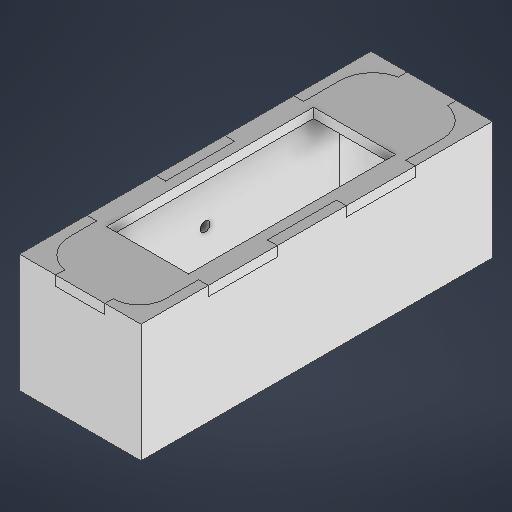
# Autodesk Inventor part: camerahouse
Saved by Autodesk Inventor 2026.2 (Build 302298000, 298)
## iProperties
Created: 2026-02-10
Part Number: camerahouse
Material: Generic
Document SubType Name: Modeling
Designer: small.ab
Density: 1 g/cm^3
Appearance: Default
Author: small.ab
Autodesk Inventor part; units mm, degrees
ref_plane "YZ Plane" through (0, 0, 0) normal (1, 0, 0) x (0, 1, 0)
ref_plane "XZ Plane" through (0, 0, 0) normal (0, 1, 0) x (-1, 0, 0)
ref_plane "XY Plane" through (0, 0, 0) normal (0, 0, 1) x (1, 0, 0)
sketch "Sketch1" plane through (0, 0, 0) normal (0, 0, 1) x (1, 0, 0)
  line L0 (0, 0) -> (100, 0)
  line L1 (100, 0) -> (100, 25)
  line L2 (100, 25) -> (0, 25)
  line L3 (0, 25) -> (0, 0)
  dimension "cameralength" = 100
  dimension "cameraheight" = 25
  constraints: 8 end point, 2 parallel, 1 horizontal, 1 perpendicular
  measures "cameralength" distance of L2.end L1.end
  measures "cameraheight" distance of L0.end L1.end
extrude "Extrusion1" add sketch "Sketch1" along normal blind 30
sketch "Sketch2" plane through (0, 0, 0) normal (0, -1, 0) x (1, 0, 0)
  line L0 (0, 0) -> (0, 30) projected
  line L1 (100, 30) -> (0, 30) projected
  line L2 (100, 0) -> (100, 30) projected
  circle A0 centre (49.9989, 14.9997) radius 9.6139
  dimension "bottomdiameter" = 19.2278
  constraints: 1 centre point
  measures "bottomdiameter" diameter of A0
extrude "Extrusion2" add sketch "Sketch2" along normal blind 5
fillet "Fillet1" radius 10 4 edges at (100, 0, 15) (100, 25, 15) (0, 0, 15) (0, 25, 15)
sketch "Sketch3" plane through (49.9989, 25, 30) normal (0, 0, 1) x (1, 0, 0)
  line L0 (53.5011, -33.5) -> (-53.4989, -33.5)
  line L1 (-53.4989, -33.5) -> (-53.4989, 3.5)
  line L2 (-53.4989, 3.5) -> (53.5011, 3.5)
  line L3 (53.5011, 3.5) -> (53.5011, -33.5)
  line L4 (53.5011, -33.5) -> (-53.4989, 3.5) construction
  line L5 (-53.4989, -33.5) -> (53.5011, 3.5) construction
  line L6 (50.0011, -25) -> (50.0011, -25) projected
  line L7 (-49.9989, -25) -> (50.0011, -25) projected
  line L8 (-49.9989, -25) -> (50.0011, -25) projected
  line L9 (50.0011, -25) -> (50.0011, -25) projected
  line L10 (-49.9989, -25) -> (50.0011, -25) projected
  line L11 (-49.9989, -25) -> (-49.9989, -25) projected
  line L12 (-42.9989, 0.5) -> (41.0011, 0.5)
  line L13 (51.0011, -9.5) -> (51.0011, -20.5)
  line L14 (41.0011, -30.5) -> (-40.9989, -30.5)
  line L15 (-50.9989, -20.5) -> (-50.9989, -7.5)
  line L16 (-50.9989, 0.5) -> (51.0011, -30.5) construction
  line L17 (51.0011, 0.5) -> (-50.9989, -30.5) construction
  line L18 (50.0011, -25) -> (50.0011, 0) projected
  line L19 (-9.6139, -30) -> (9.6139, -30) projected
  line L20 (9.6139, -25) -> (-9.6139, -25) projected
  line L21 (50.0011, 0) -> (-49.9989, 0) projected
  arc A0 (-50.9989, -20.5) -> (-40.9989, -30.5) centre (-40.9989, -20.5) ccw
  arc A1 (-42.9989, 0.5) -> (-50.9989, -7.5) centre (-42.9989, -7.5) ccw
  arc A2 (41.0011, -30.5) -> (51.0011, -20.5) centre (41.0011, -20.5) ccw
  arc A3 (51.0011, -9.5) -> (41.0011, 0.5) centre (41.0011, -9.5) ccw
  point P0 (0.0011, -15)
  point P1 (50.0011, 15.0003)
  point P2 (-49.9989, -14.9997)
  point P3 (44.1236, 0)
  point P4 (50.0011, -5.1411)
  point P5 (50.0011, -24.8589)
  point P6 (49.9314, -25)
  dimension "d7" = 37
  dimension "d8" = 107
  dimension "d9" = 3.5
  dimension "d16" = 1
  dimension "d18" = 0.5
  dimension "d19" = 31
  dimension "d20" = 3
  dimension "fillet" = 10
  dimension "d25" = 8
  dimension "d26" = 10
  dimension "d27" = 10
  constraints: 24 end point, 8 point on circle, 8 point on line, 8 tangent, 4 centre point, 4 midpoint, 4 parallel, 2 horizontal, 2 perpendicular
  measures "d7" distance between parallel lines of L0 L2
  measures "d8" distance between parallel lines of L3 L1
  measures "d9" distance between parallel lines of L3 L6
  measures "d16" distance between parallel lines of L13 L18
  measures "d18" distance between parallel lines of L12 L21
  measures "d19" distance between parallel lines of L12 L14
  measures "d20" distance between parallel lines of L14 L0
  measures "fillet" radius of A0
  measures "d25" radius of A1
  measures "d26" radius of A2
  measures "d27" radius of A3
extrude "Extrusion3" add sketch "Sketch3" against normal blind 33 separate body contours L0 L1 L2 L3 | A3 L21 L18
sketch "Sketch4" plane through (49.9989, 25, 30) normal (0, 0, 1) x (1, 0, 0)
  line L0 (53.5011, 3.5) -> (-53.4989, 3.5) projected
  line L1 (-53.4989, 3.5) -> (-53.4989, -33.5) projected
  line L2 (-53.4989, -33.5) -> (53.5011, -33.5) projected
  line L3 (53.5011, -33.5) -> (53.5011, 3.5) projected
  line L4 (-42.9989, 0.5) -> (41.0011, 0.5) projected
  line L5 (51.0011, -9.5) -> (51.0011, -20.5) projected
  line L6 (41.0011, -30.5) -> (-40.9989, -30.5) projected
  line L7 (-50.9989, -20.5) -> (-50.9989, -7.5) projected
  line L8 (-53.4989, 3.5) -> (53.5011, 3.5)
  line L9 (53.5011, 3.5) -> (53.5011, -33.5)
  line L10 (53.5011, -33.5) -> (-53.4989, -33.5)
  line L11 (-53.4989, -33.5) -> (-53.4989, 3.5)
  circle A0 centre (0.0011, -12.5) radius 10
  line L12 (50.0011, -15) -> (50.0011, -10) projected
  line L13 (40.0011, 0) -> (-39.9989, 0) projected
  line L14 (-49.9989, -10) -> (-49.9989, -15) projected
  line L15 (-39.9989, -25) -> (40.0011, -25) projected
  arc A1 (51.0011, -9.5) -> (41.0011, 0.5) centre (41.0011, -9.5) ccw projected
  line L16 (50.0011, -24.8589) -> (50.0011, -25) projected
  arc A2 (50.0011, -24.8589) -> (51.0011, -20.5) centre (41.0011, -20.5) ccw projected
  line L17 (50.0011, -25) -> (49.9314, -25) projected
  arc A3 (41.0011, -30.5) -> (49.9314, -25) centre (41.0011, -20.5) ccw projected
  arc A4 (-50.9989, -20.5) -> (-40.9989, -30.5) centre (-40.9989, -20.5) ccw projected
  arc A5 (-42.9989, 0.5) -> (-50.9989, -7.5) centre (-42.9989, -7.5) ccw projected
  arc A6 (-39.9989, 0) -> (-49.9989, -10) centre (-39.9989, -10) ccw projected
  arc A7 (-49.9989, -15) -> (-39.9989, -25) centre (-39.9989, -15) ccw projected
  arc A8 (40.0011, -25) -> (50.0011, -15) centre (40.0011, -15) ccw projected
  arc A9 (50.0011, -10) -> (40.0011, 0) centre (40.0011, -10) ccw projected
  point P0 (-49.9989, -25)
  dimension "cordhole" = 20
  constraints: 8 end point, 2 parallel, 1 centre point, 1 horizontal, 1 perpendicular
  measures "cordhole" diameter of A0
extrude "Extrusion4" add sketch "Sketch4" along normal blind 3 contours L3 L2 L1 L0 | L4 A1 L5 A2 L16 L17 A3 L6 A4 L7 A5 | A8 L15 A7 L14 A6 L13 A9 L12 bodies 2
sketch "Sketch5" plane through (-3.5, -8.5, 0) normal (0, -1, 0) x (1, 0, 0)
  circle A0 centre (53.4989, 14.9997) radius 9.6139 projected
  circle A1 centre (53.4989, 14.9997) radius 1.5
  point P0 (3.5, 0)
  dimension "screwdiameter" = 3
  constraints: 1 centre point, 1 coincident
  measures "screwdiameter" diameter of A1
extrude "Extrusion5" cut sketch "Sketch5" against normal blind 3 contours A1 bodies 2
sketch "Sketch7" plane through (-3.5, 28.5, 0) normal (0, 1, 0) x (1, 0, 0)
  line L0 (0, 3) -> (0, -33) projected
  line L1 (107, -33) -> (0, -33) projected
  line L2 (107, -33) -> (107, 3) projected
  line L3 (104.5, -30) -> (104.5, 3) projected
  line L4 (2.5, -30) -> (2.5, 3) projected
  line L5 (104.5, 0) -> (2.5, 0)
  line L6 (2.5, 0) -> (2.5, 0)
  line L7 (2.5, 0) -> (104.5, 0)
  line L8 (104.5, 0) -> (104.5, 0)
  line L9 (83.5, 0) -> (83.5, 0)
  line L10 (62.5, 0) -> (62.5, 0)
  line L11 (41.5, -3) -> (41.5, 0)
  line L12 (20.5, -3) -> (20.5, 0)
  line L13 (0, 3) -> (107, 3) projected
  line L14 (83.5, 0) -> (83.5, 3)
  line L15 (62.5, 0) -> (62.5, 3)
  line L16 (41.5, 0) -> (41.5, 3)
  line L17 (20.5, 0) -> (20.5, 3)
  line L18 (0, 3) -> (107, 3) projected
  point P0 (3.5, 0)
  point P1 (20.5, 0)
  point P2 (41.5, 0)
  point P3 (62.5, -3)
  point P4 (20.5, 0)
  point P5 (62.5, 0)
  point P6 (41.5, 0)
  point P7 (20.5, 0)
  point P8 (41.5, 0)
  dimension "d44" = 21
  dimension "d47" = 21
  dimension "d59" = 3
  constraints: 24 end point, 7 point on line, 5 perpendicular, 2 equal length, 1 horizontal
  measures "d44" distance between parallel lines of L9 L3
  measures "d47" distance of L9.start L10.start
  measures "d59" distance between parallel lines of L13 L7
extrude "Extrusion9" cut sketch "Sketch7" against normal up to surface (37 mm away) contours L13 L16 L5 L17 | L13 L14 L5 L15 bodies 2
sketch "Sketch8" plane through (103.5, -8.5, 0) normal (1, 0, 0) x (0, 0, -1)
  line L0 (-33, 37) -> (3, 37) projected
  line L1 (-33, 0) -> (-33, 37) projected
  line L2 (3, 0) -> (-33, 0) projected
  line L3 (-30, 3) -> (3, 3) projected
  line L4 (-30, 34) -> (3, 34) projected
  line L5 (3, 37) -> (3, 0) projected
  line L6 (3, 37) -> (0, 37)
  line L7 (0, 37) -> (0, 0)
  line L8 (0, 0) -> (3, 0)
  line L9 (3, 0) -> (3, 37)
  line L10 (0, 26) -> (3, 26)
  line L11 (0, 11) -> (3, 11)
  line L12 (3, 13) -> (3, 8.6411) projected
  point P0 (-3, 34)
  point P1 (0, 3)
  dimension "d62" = 11
  dimension "d63" = 11
  constraints: 12 end point, 5 point on line, 3 parallel, 2 perpendicular, 1 horizontal
  measures "d62" distance between parallel lines of L2 L11
  measures "d63" distance from line of L10 L0.end
extrude "Extrusion10" cut sketch "Sketch8" against normal up to surface (107 mm away) contours L10 L5 L11 L7 bodies 2
sketch "Sketch11" plane through (49.9989, 25, -3) normal (0, 0, -1) x (-1, 0, 0)
  line L0 (-53.5011, -7.5) -> (-50.7991, -7.5) projected
  arc A0 (-41.0011, 0.5) -> (-50.7991, -7.5) centre (-41.0011, -9.5) ccw projected
  line L1 (-41.0011, 0.5) -> (-30.0011, 0.5) projected
  line L2 (-30.0011, 0.5) -> (-30.0011, 3.5) projected
  line L3 (-30.0011, 3.5) -> (-53.5011, 3.5) projected
  line L4 (-53.5011, 3.5) -> (-53.5011, -7.5) projected
  line L5 (-53.5011, -22.5) -> (-53.5011, -7.5) projected
  arc A1 (-51.0011, -20.5) -> (-50.7991, -22.5) centre (-41.0011, -20.5) ccw projected
  line L6 (-51.0011, -9.5) -> (-51.0011, -20.5) projected
  arc A2 (-50.7991, -7.5) -> (-51.0011, -9.5) centre (-41.0011, -9.5) ccw projected
  line L7 (-53.5011, -7.5) -> (-50.7991, -7.5) projected
  line L8 (-53.5011, -22.5) -> (-53.5011, -7.5) projected
  line L9 (-53.5011, -22.5) -> (-50.7991, -22.5) projected
  line L10 (-50.7991, -22.5) -> (-53.5011, -22.5) projected
  line L11 (-53.5011, -22.5) -> (-53.5011, -33.5) projected
  line L12 (-53.5011, -33.5) -> (-30.0011, -33.5) projected
  line L13 (-30.0011, -33.5) -> (-30.0011, -30.5) projected
  line L14 (-30.0011, -30.5) -> (-41.0011, -30.5) projected
  arc A3 (-49.9314, -25) -> (-41.0011, -30.5) centre (-41.0011, -20.5) ccw projected
  line L15 (-49.9314, -25) -> (-50.0011, -25) projected
  line L16 (-50.0011, -25) -> (-50.0011, -24.8589) projected
  arc A4 (-50.7991, -22.5) -> (-50.0011, -24.8589) centre (-41.0011, -20.5) ccw projected
  line L17 (-30.0011, -30.5) -> (-9.0011, -30.5) projected
  line L18 (-30.0011, -30.5) -> (-30.0011, -33.5) projected
  line L19 (-9.0011, -33.5) -> (-30.0011, -33.5) projected
  line L20 (-9.0011, -30.5) -> (-9.0011, -33.5) projected
  line L21 (-9.0011, 0.5) -> (-30.0011, 0.5) projected
  line L22 (-9.0011, 3.5) -> (-9.0011, 0.5) projected
  line L23 (-30.0011, 3.5) -> (-9.0011, 3.5) projected
  line L24 (-30.0011, 3.5) -> (-30.0011, 0.5) projected
  line L25 (11.9989, 0.5) -> (11.9989, 3.5) projected
  line L26 (11.9989, 3.5) -> (-9.0011, 3.5) projected
  line L27 (-9.0011, 3.5) -> (-9.0011, 0.5) projected
  line L28 (-9.0011, 0.5) -> (11.9989, 0.5) projected
  line L29 (11.9989, -33.5) -> (11.9989, -30.5) projected
  line L30 (11.9989, -30.5) -> (-9.0011, -30.5) projected
  line L31 (-9.0011, -30.5) -> (-9.0011, -33.5) projected
  line L32 (-9.0011, -33.5) -> (11.9989, -33.5) projected
  line L33 (11.9989, -30.5) -> (32.9989, -30.5) projected
  line L34 (11.9989, -30.5) -> (11.9989, -33.5) projected
  line L35 (32.9989, -33.5) -> (11.9989, -33.5) projected
  line L36 (32.9989, -30.5) -> (32.9989, -33.5) projected
  line L37 (32.9989, 0.5) -> (11.9989, 0.5) projected
  line L38 (32.9989, 3.5) -> (32.9989, 0.5) projected
  line L39 (11.9989, 3.5) -> (32.9989, 3.5) projected
  line L40 (11.9989, 3.5) -> (11.9989, 0.5) projected
  line L41 (50.9989, -7.5) -> (53.4989, -7.5) projected
  line L42 (53.4989, -7.5) -> (53.4989, 3.5) projected
  line L43 (53.4989, 3.5) -> (32.9989, 3.5) projected
  line L44 (32.9989, 3.5) -> (32.9989, 0.5) projected
  line L45 (32.9989, 0.5) -> (42.9989, 0.5) projected
  arc A5 (50.9989, -7.5) -> (42.9989, 0.5) centre (42.9989, -7.5) ccw projected
  line L46 (50.9989, -20.5) -> (50.9989, -7.5) projected
  arc A6 (50.7969, -22.5) -> (50.9989, -20.5) centre (40.9989, -20.5) ccw projected
  line L47 (50.7969, -22.5) -> (53.4989, -22.5) projected
  line L48 (53.4989, -7.5) -> (53.4989, -22.5) projected
  line L49 (50.9989, -7.5) -> (53.4989, -7.5) projected
  line L50 (53.4989, -22.5) -> (50.7969, -22.5) projected
  arc A7 (40.9989, -30.5) -> (50.7969, -22.5) centre (40.9989, -20.5) ccw projected
  line L51 (40.9989, -30.5) -> (32.9989, -30.5) projected
  line L52 (32.9989, -30.5) -> (32.9989, -33.5) projected
  line L53 (32.9989, -33.5) -> (53.4989, -33.5) projected
  line L54 (53.4989, -33.5) -> (53.4989, -22.5) projected
  line L55 (-53.5011, 3.5) -> (53.4989, 3.5)
  line L56 (53.4989, 3.5) -> (53.4989, -33.5)
  line L57 (53.4989, -33.5) -> (-53.5011, -33.5)
  line L58 (-53.5011, -33.5) -> (-53.5011, 3.5)
  line L59 (-30.0011, 0.5) -> (-30.0011, -30.5)
  line L60 (32.9989, 0.5) -> (32.9989, -30.5)
  line L61 (-30.0011, -2.5) -> (32.9989, -2.5)
  line L62 (32.9989, -27.5) -> (-30.0011, -27.5)
  point P0 (49.9989, -25)
  dimension "d70" = 3
  dimension "d71" = 3
  constraints: 16 end point, 4 point on line, 3 perpendicular, 2 parallel, 1 horizontal, 1 vertical
  measures "d70" distance between parallel lines of L21 L61
  measures "d71" distance between parallel lines of L17 L62
extrude "Extrusion12" add sketch "Sketch11" against normal blind 3 separate body contours L0 A2 L6 A1 L9 L5 | A0 L1 L59 L14 A3 L15 L16 A4 A1 L6 A2 | L23 L22 L21 L2 | L21 L28 L37 L60 L61 L59 | L13 L17 L20 L19 | L39 L38 L37 L25 | L59 L62 L60 L33 L30 L17 | L60 L45 A5 L46 A6 A7 L51 | L29 L33 L36 L35 | L48 L47 A6 L46 L41
equation "\"d28\" = fillet"
equation "\"d7\" = 2 * wallthickness + cameraheight + bottomheight + tolerance"
equation "\"d8\" = 2 * wallthickness + cameralength + tolerance"
equation "\"d9\" = wallthickness + 0.5 * tolerance"
equation "\"d16\" = tolerance"
equation "\"d18\" = 0.5 * tolerance"
equation "\"d19\" = bottomheight + cameraheight + tolerance"
equation "\"d11\" = camerawidth + wallthickness"
equation "\"d22\" = wallthickness"
equation "\"d30\" = wallthickness"
equation "\"d59\" = wallthickness"
equation "\"d70\" = wallthickness"
equation "\"d71\" = wallthickness"
equation "\"d68\" = wallthickness"
equation "\"tolerance\" = 1"
equation "\"wallthickness\" = 3"
equation "\"bottomheight\" = 5"
equation "\"camerawidth\" = 30"
body "Solid4"
